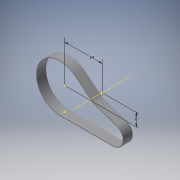
# Autodesk Inventor part: PasekBaza
Saved by Autodesk Inventor 2019 (Build 230136000, 136)
## iProperties
Created: 2020-08-21
Part Number: PasekBaza
Material: Generic
Document SubType Name: Modeling
Designer: estee
Density: 1 g/cm^3
Appearance: Default
Author: estee
Autodesk Inventor part; units mm, degrees
ref_plane "XZ Plane" through (0, 0, 0) normal (0, 1, 0) x (-1, 0, 0)
ref_plane "Work Plane1" through (34, 0, 0) normal (-1, 0, 0) x (0, 1, 0)
ref_plane "Work Plane2" through (24, 0, 0) normal (-1, 0, 0) x (0, 1, 0)
sketch "Sketch1" plane through (0, 0, 0) normal (0, 0, 1) x (1, 0, 0)
  arc A0 (9.4163, 11.6454) -> (0, -14.976) centre (0, 0) ccw
  arc A1 (34, -14.976) -> (36.0136, -2.7599) centre (34, -8.702) ccw
  line L0 (-31.8369, 0) -> (53.8728, 0) construction
  line L1 (0, -14.976) -> (34, -14.976)
  arc A2 (20.0168, 3.0739) -> (21.9668, 2.0001) centre (24, 8) ccw
  line L2 (9.4163, 11.6454) -> (20.0168, 3.0739)
  line L3 (21.9668, 2.0001) -> (36.0136, -2.7599)
  line L4 (0, 26.7627) -> (0, -23.4277) construction
  line L5 (34, -23.4277) -> (34, 26.7627) construction
  line L6 (24, -23.4277) -> (24, 26.7627) construction
  arc A3 (9.6527, 11.9377) -> (0, -15.352) centre (0, 0) ccw
  line L7 (9.6527, 11.9377) -> (20.2532, 3.3663)
  arc A4 (20.2532, 3.3663) -> (22.0875, 2.3562) centre (24, 8) ccw
  line L8 (22.0875, 2.3562) -> (36.1343, -2.4038)
  arc A5 (34, -15.352) -> (36.1343, -2.4038) centre (34, -8.702) ccw
  line L9 (34, -15.352) -> (0, -15.352)
  dimension "d1" = 29.952
  dimension "d2" = 12.548
  dimension "d3" = 34
  dimension "d4" = 8.702
  dimension "d6" = 12.67
  dimension "d7" = 24
  dimension "d8" = 8
  dimension "d9" = 34
  dimension "d10" = 24
  dimension "d16" = 0.376
  constraints: 12 end point, 12 point on circle, 6 centre point, 5 tangent, 2 coincident, 1 horizontal, 5 other
  measures "d1" diameter of A0
  measures "d2" diameter of A1
  measures "d3" horizontal distance of A1.centre A0.centre
  measures "d4" distance from line of L0 A1.centre
  measures "d6" diameter of A2
  measures "d7" horizontal distance of A2.centre point (0, 0)
  measures "d8" distance from line of L0 A2.centre
  measures "d9" distance between parallel lines of L5 L4
  measures "d10" distance between parallel lines of L6 L4
  measures "d16" radial gap between concentric circles of A0 A3
extrude "Extrusion1" add sketch "Sketch1" along normal mid plane 6
sketch "Sketch2" plane through (0, 0, 0) normal (0, 0, 1) x (1, 0, 0)
  point P0 (0, 0)
  point P1 (24, 8)
  dimension "d19" = 24
  dimension "d20" = 8
  measures "d19" horizontal distance of point (0, 0) point (24, 8)
  measures "d20" vertical distance of point (0, 0) point (24, 8)
equation "\"start\" = d9"
body "Solid1"
